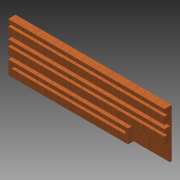
# Autodesk Inventor part: ply75_bottom_board
Saved by Autodesk Inventor 2014 SP1 (Build 180222100, 222)
## iProperties
Created: 2014-02-20
Part Number: ply75_bottom_board
Material: Wood (Cherry)
Document SubType Name: Modeling
Designer: Chris
Density: 0.63 g/cm^3
Appearance: Cherry - Natural Low Gloss
Mass: 1132.99 g
Surface Area: 2808.87 cm^2
Volume: 1798.4 cm^3
Author: Chris
Autodesk Inventor part; units mm, degrees
ref_plane "YZ Plane" through (0, 0, 0) normal (1, 0, 0) x (0, 1, 0)
ref_plane "XZ Plane" through (0, 0, 0) normal (0, 1, 0) x (-1, 0, 0)
sketch "Sketch1" plane through (0, 0, 0) normal (0, 0, 1) x (1, 0, 0)
  line L0 (0, 0) -> (539.75, 0)
  line L1 (539.75, 0) -> (539.75, 168.275)
  line L2 (539.75, 168.275) -> (0, 168.275)
  line L3 (0, 168.275) -> (0, 0)
  dimension "d0" = 539.75
  dimension "d1" = 168.275
  constraints: 8 end point, 2 parallel, 1 horizontal, 1 perpendicular
  measures "d0" distance of L1.end L2.end
  measures "d1" distance of L2.end L0.start
extrude "Extrusion1" add sketch "Sketch1" along normal blind 25.4
sketch "Sketch2" plane through (0, 0, 25.4) normal (0, 0, 1) x (1, 0, 0)
  line L0 (539.75, 0) -> (539.75, 168.275) projected
  line L1 (0, 168.275) -> (0, 0) projected
  line L2 (0, 168.275) -> (539.75, 168.275)
  line L3 (539.75, 168.275) -> (539.75, 120.65)
  line L4 (539.75, 120.65) -> (0, 120.65)
  line L5 (0, 120.65) -> (0, 168.275)
  line L6 (0, 107.95) -> (539.75, 107.95)
  line L7 (539.75, 107.95) -> (539.75, 60.325)
  line L8 (539.75, 60.325) -> (0, 60.325)
  line L9 (0, 60.325) -> (0, 107.95)
  line L10 (0, 47.625) -> (539.75, 47.625)
  line L11 (539.75, 47.625) -> (539.75, 0)
  line L12 (539.75, 0) -> (0, 0)
  line L13 (0, 0) -> (0, 47.625)
  line L14 (0, 120.65) -> (539.75, 120.65)
  line L15 (539.75, 120.65) -> (539.75, 107.95)
  line L16 (539.75, 107.95) -> (0, 107.95)
  line L17 (0, 107.95) -> (0, 120.65)
  line L18 (539.75, 60.325) -> (0, 60.325)
  line L19 (0, 60.325) -> (0, 47.625)
  line L20 (0, 47.625) -> (539.75, 47.625)
  line L21 (539.75, 47.625) -> (539.75, 60.325)
  dimension "d4" = 47.625
  dimension "d5" = 47.625
  dimension "d6" = 47.625
  dimension "d7" = 12.7
  dimension "d8" = 12.7
  constraints: 40 end point, 10 parallel, 5 horizontal, 5 perpendicular, 4 point on line
  measures "d4" distance of L2.end L3.end
  measures "d5" distance of L10.end L0.start
  measures "d6" distance between parallel lines of L8 L6
  measures "d7" distance between parallel lines of L6 L4
  measures "d8" distance between parallel lines of L10 L8
extrude "Extrusion3" cut sketch "Sketch2" against normal blind 19.05 contours L10 L1 L8 L0 | L6 L1 L4 L0
sketch "Sketch3" plane through (0, 0, 25.4) normal (0, 0, 1) x (1, 0, 0)
  line L0 (0, 120.65) -> (539.75, 120.65) projected
  line L1 (539.75, 120.65) -> (539.75, 168.275) projected
  line L2 (539.75, 168.275) -> (0, 168.275) projected
  line L3 (0, 168.275) -> (0, 120.65) projected
  line L4 (0, 155.575) -> (539.75, 155.575)
  line L5 (539.75, 155.575) -> (539.75, 146.05)
  line L6 (539.75, 146.05) -> (0, 146.05)
  line L7 (0, 146.05) -> (0, 155.575)
  line L8 (0, 107.95) -> (558.8, 107.95)
  line L9 (558.8, 107.95) -> (558.8, 60.325)
  line L10 (558.8, 60.325) -> (0, 60.325)
  line L11 (0, 60.325) -> (0, 107.95)
  line L12 (1.6074, 47.625) -> (558.8, 47.625)
  line L13 (558.8, 47.625) -> (558.8, 0)
  line L14 (558.8, 0) -> (1.6074, 0)
  line L15 (1.6074, 0) -> (1.6074, 47.625)
  line L16 (0, 95.25) -> (558.8, 95.25)
  line L17 (558.8, 95.25) -> (558.8, 85.725)
  line L18 (558.8, 85.725) -> (0, 85.725)
  line L19 (0, 85.725) -> (0, 95.25)
  line L20 (11.1324, 34.925) -> (404.8324, 34.925)
  line L21 (404.8324, 34.925) -> (404.8324, 25.4)
  line L22 (404.8324, 25.4) -> (11.1324, 25.4)
  line L23 (11.1324, 25.4) -> (11.1324, 34.925)
  line L24 (558.8, 47.625) -> (414.3574, 47.625)
  line L25 (414.3574, 47.625) -> (414.3574, 0)
  line L26 (414.3574, 0) -> (558.8, 0)
  line L27 (558.8, 0) -> (558.8, 47.625)
  point P0 (0, 0)
  dimension "d13" = 9.525
  dimension "d14" = 12.7
  dimension "d15" = 25.4
  dimension "d16" = 12.7
  dimension "d17" = 12.7
  dimension "d18" = 47.625
  dimension "d19" = 47.625
  dimension "d20" = 9.525
  dimension "d21" = 12.7
  dimension "d22" = 393.7
  dimension "d23" = 412.75
  dimension "d24" = 9.525
  dimension "d25" = 9.525
  dimension "d26" = 9.525
  dimension "d27" = 12.7
  dimension "d28" = 539.75
  constraints: 48 end point, 12 parallel, 6 horizontal, 6 perpendicular, 5 point on line
  measures "d13" distance between parallel lines of L6 L4
  measures "d14" distance between parallel lines of L2 L4
  measures "d15" distance between parallel lines of L0 L6
  measures "d16" distance between parallel lines of L8 L0
  measures "d17" distance between parallel lines of L12 L10
  measures "d18" distance of L8.end L9.end
  measures "d19" distance of L12.end L13.end
  measures "d20" distance between parallel lines of L18 L16
  measures "d21" distance between parallel lines of L16 L8
  measures "d22" distance of L20.start L20.end
  measures "d23" distance between parallel lines of L25 L15
  measures "d24" distance between parallel lines of L25 L21
  measures "d25" distance between parallel lines of L15 L23
  measures "d26" distance between parallel lines of L22 L20
  measures "d27" distance between parallel lines of L12 L20
  measures "d28" distance of L1.end L2.end
ref_plane "Work Plane1" through (0, 0, 15.875) normal (0, 0, 1) x (1, 0, 0)
sketch "Sketch5" plane through (0, 0, 15.875) normal (0, 0, 1) x (1, 0, 0)
  line L0 (539.75, 47.625) -> (539.75, 0) projected
  line L1 (414.3574, 47.625) -> (539.75, 47.625) projected
  line L2 (414.3574, 0) -> (414.3574, 47.625) projected
  line L3 (539.75, 0) -> (414.3574, 0) projected
  point P0 (0, 0)
extrude "Extrusion5" cut sketch "Sketch5" against normal blind 9.525
extrude "Extrusion7" cut sketch "Sketch3" against normal blind 9.525 contours L3 L4 L1 L6 | L16 L9 L18 L11 | L12 L13 L14 L25 | L20 L21 L22 L23
equation "\"d7\" = d8"
equation "\"d19\" = d18"
equation "\"d24\" = d25"
body "Solid1"
